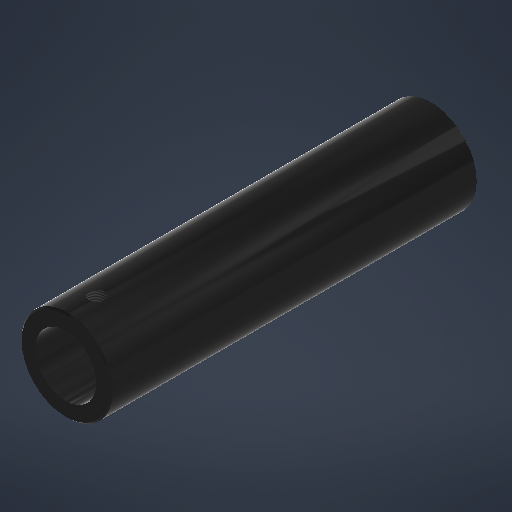
# Autodesk Inventor part: stand_base
Saved by Autodesk Inventor 2026 (Build 300175050, 175E)
## iProperties
Created: 2025-07-09
Part Number: stand_base
Material: UHMW、黒
Document SubType Name: Modeling
Designer: jin20
Density: 0.94 g/cm^3
Appearance: 滑らか - 黒
Author: jin20
Autodesk Inventor part; units mm, degrees
ref_plane "YZ Plane" through (0, 0, 0) normal (1, 0, 0) x (0, 1, 0)
ref_plane "XZ Plane" through (0, 0, 0) normal (0, 1, 0) x (-1, 0, 0)
ref_plane "XY Plane" through (0, 0, 0) normal (0, 0, 1) x (1, 0, 0)
sketch "スケッチ1" plane through (0, 0, 0) normal (0, 1, 0) x (-1, 0, 0)
  line L0 (-5.0796, -45.5704) -> (-5.0796, 73.9296)
  line L1 (-5.0796, 73.9296) -> (-4.5796, 74.4296)
  line L2 (-4.5796, 74.4296) -> (24.4204, 74.4296)
  line L3 (24.4204, 74.4296) -> (24.9204, 73.9296)
  line L4 (24.9204, 73.9296) -> (24.9204, -45.5704)
  line L5 (24.9204, -45.5704) -> (-5.0796, -45.5704)
  line L6 (1.9204, -47.0704) -> (1.9204, -50.5704)
  line L7 (1.9204, -50.5704) -> (17.9204, -50.5704)
  line L8 (17.9204, -50.5704) -> (17.9204, -47.0704)
  line L9 (17.9204, -47.0704) -> (1.9204, -47.0704)
  line L10 (2.9204, -47.0704) -> (2.9204, -45.5704)
  line L11 (16.9204, -45.5704) -> (16.9204, -47.0704)
  line L12 (31.4204, 56.4296) -> (30.9204, 56.9296)
  line L13 (30.9204, 56.9296) -> (30.9204, 71.9296)
  line L14 (30.9204, 71.9296) -> (31.4204, 72.4296)
  line L15 (31.4204, 72.4296) -> (38.4204, 72.4296)
  line L16 (38.4204, 72.4296) -> (38.9204, 71.9296)
  line L17 (38.9204, 71.9296) -> (38.9204, 56.9296)
  line L18 (38.9204, 56.9296) -> (38.4204, 56.4296)
  line L19 (38.4204, 56.4296) -> (31.4204, 56.4296)
  line L20 (31.4204, 56.4296) -> (31.4204, 72.4296)
  line L21 (30.9204, 70.4296) -> (27.9204, 70.4296)
  line L22 (27.9204, 70.4296) -> (27.9204, 58.4296)
  line L23 (27.9204, 58.4296) -> (30.9204, 58.4296)
  line L24 (38.4204, 56.4296) -> (38.4204, 72.4296)
  line L25 (27.9204, 66.9296) -> (24.9204, 66.9296)
  line L26 (27.4204, 66.9296) -> (27.4204, 61.9296)
  line L27 (27.9204, 61.9296) -> (24.9204, 61.9296)
  line L28 (24.9204, 73.9296) -> (-5.0796, 73.9296)
  line L29 (-5.0796, 97.1797) -> (24.9204, 97.1797)
  line L30 (24.9204, 97.1797) -> (24.9204, 105.1797)
  line L31 (24.9204, 105.1797) -> (-5.0796, 105.1797)
  line L32 (-5.0796, 105.1797) -> (-5.0796, 97.1797)
  line L33 (24.9204, 99.1797) -> (27.9204, 99.1797)
  line L34 (27.2723, 99.1797) -> (27.2723, 103.1797)
  line L35 (27.9204, 103.1797) -> (24.9204, 103.1797)
  line L36 (27.9204, 105.6797) -> (27.9204, 96.6797)
  line L37 (27.9204, 96.6797) -> (28.4204, 96.1797)
  line L38 (28.4204, 96.1797) -> (32.4204, 96.1797)
  line L39 (32.4204, 96.1797) -> (32.9204, 96.6797)
  line L40 (32.9204, 96.6797) -> (32.9204, 105.6797)
  line L41 (32.9204, 105.6797) -> (32.4204, 106.1797)
  line L42 (32.4204, 106.1797) -> (28.4204, 106.1797)
  line L43 (28.4204, 106.1797) -> (27.9204, 105.6797)
  line L44 (28.4204, 106.1797) -> (28.4204, 96.1797)
  line L45 (32.4204, 96.1797) -> (32.4204, 106.1797)
  line L46 (2.4204, -50.5704) -> (2.4204, -47.0704)
  line L47 (-0.0796, -40.5704) -> (-0.0796, 74.4296)
  line L48 (19.9204, 74.4296) -> (19.9204, -40.5704)
  line L49 (19.9204, -40.5704) -> (9.9204, -46.3439)
  line L50 (9.9204, -46.3439) -> (-0.0796, -40.5704)
  line L51 (-0.0796, -40.5704) -> (19.9204, -40.5704)
  line L52 (17.4204, -47.0704) -> (17.4204, -50.5704)
  line L53 (9.9204, -56.5156) -> (9.9204, 78.76)
  line L54 (9.9204, 93.5864) -> (9.9204, 108.5157)
  line L55 (19.9204, 105.1797) -> (19.9204, 97.1797)
  line L56 (22.5096, 101.1797) -> (35.2156, 101.1797)
  line L57 (27.9204, 103.1797) -> (27.2723, 102.4797)
  line L58 (27.2723, 102.4797) -> (24.9204, 102.4797)
  line L59 (24.9204, 99.8797) -> (27.2723, 99.8797)
  line L60 (27.2723, 99.8797) -> (27.9204, 99.1797)
  line L61 (-0.0796, 97.1797) -> (-0.0796, 105.1797)
  line L62 (24.9204, 66.2296) -> (27.4204, 66.2296)
  line L63 (27.4204, 66.2296) -> (27.9204, 66.9296)
  line L64 (27.4204, 62.6296) -> (27.9204, 61.9296)
  line L65 (27.4204, 62.6296) -> (24.9204, 62.6296)
  line L66 (22.6428, 64.4296) -> (42.5049, 64.4296)
  line L67 (32.2954, 71.4296) -> (38.4204, 71.4296)
  line L68 (33.1704, 70.4296) -> (38.4204, 70.4296)
  line L69 (34.0454, 69.4296) -> (38.4204, 69.4296)
  line L70 (34.9204, 68.4296) -> (38.4204, 68.4296)
  line L71 (35.7954, 67.4296) -> (38.4204, 67.4296)
  line L72 (36.6704, 66.4296) -> (38.4204, 66.4296)
  line L73 (37.5454, 65.4296) -> (38.4204, 65.4296)
  line L74 (29.2204, 105.1797) -> (32.4204, 105.1797)
  line L75 (30.0204, 104.1797) -> (32.4204, 104.1797)
  line L76 (30.8204, 103.1797) -> (32.4204, 103.1797)
  line L77 (31.6204, 102.1797) -> (32.4204, 102.1797)
  point P0 (0, 0)
  point P1 (52.3578, -69.094)
  point P2 (52.3578, -59.2279)
  point P3 (9.9204, 74.4296)
  point P4 (9.9204, -45.5704)
  point P5 (11.2601, -45.5704)
  point P6 (9.9204, -46.3439)
  point P7 (9.9204, -50.5704)
  point P8 (24.4204, 74.4296)
  constraints: 156 end point, 2 other
revolve "回転1" add sketch "スケッチ1" angle 360 about axis through (-9.9204, 0, -56.5156) along (0, 0, 1) contours L49 L5 L11 L9 L53 | L9 L52 L7 L53 | L48 L2 L3 L28 | L28 L4 L5 L49 L48 | L9 L8 L7 L52
sketch "スケッチ2" plane through (-9.9204, 0, 74.4296) normal (0, 0, 1) x (1, 0, 0)
  line L0 (0, 0) -> (55.7189, 0) construction
  point P0 (9.9204, 0)
  constraints: 2 end point, 1 horizontal
ref_plane "作業平面1" through (-9.9204, 0, 74.4296) normal (0, -1, 0) x (1, 0, 0)
sketch "スケッチ3" plane through (-9.9204, 0, 74.4296) normal (0, -1, 0) x (1, 0, 0)
  line L0 (10, 0) -> (-10, 0) projected
  line L1 (0, 0) -> (0, -10) construction
  circle A0 centre (0, -10) radius 2.5
  point P0 (9.9204, -74.4296)
  dimension "d2" = 10
  dimension "d3" = 5
  constraints: 2 end point, 1 centre point, 1 coincident, 1 midpoint, 1 vertical
  measures "d2" distance of L1.start L1.end
  measures "d3" diameter of A0
extrude "押し出し1" cut sketch "スケッチ3" against normal through all
thread "ねじ1" size "M5x0.8" class "6H" standard "ANSI Metric M Profile" full length
thread "ねじ2" size "M16x2" class "6g" standard "ANSI Metric M Profile" full length
